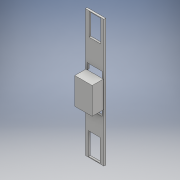
# Autodesk Inventor part: Base_trem
Saved by Autodesk Inventor 2018 (Build 220112000, 112)
## iProperties
Created: 2018-02-24
Part Number: Base_trem
Material: Generic
Document SubType Name: Modeling
Designer: matheus
Density: 1 g/cm^3
Appearance: Default
Author: matheus
Autodesk Inventor part; units mm, degrees
ref_plane "YZ Plane" through (0, 0, 0) normal (1, 0, 0) x (0, 1, 0)
ref_plane "XZ Plane" through (0, 0, 0) normal (0, 1, 0) x (-1, 0, 0)
ref_plane "XY Plane" through (0, 0, 0) normal (0, 0, 1) x (1, 0, 0)
sketch "Sketch1" plane through (0, 0, 0) normal (0, 1, 0) x (-1, 0, 0)
  line L0 (-15, 102.5) -> (15, 102.5)
  line L1 (15, 102.5) -> (15, -102.5)
  line L2 (15, -102.5) -> (-15, -102.5)
  line L3 (-15, -102.5) -> (-15, 102.5)
  point P0 (0, 0)
  constraints: 8 end point, 2 parallel, 1 horizontal, 1 perpendicular
extrude "Extrusion1" add sketch "Sketch1" along normal blind 3
sketch "Sketch2" plane through (0, 0, 0) normal (0, -1, 0) x (1, 0, 0)
  line L0 (-15, -102.5) -> (-15, 102.5) projected
  line L1 (-15, -102.5) -> (-15, -101.5)
  line L2 (-10, -101.5) -> (9, -101.5)
  line L3 (9, -101.5) -> (9, -65.5)
  line L4 (9, -65.5) -> (-10, -65.5)
  line L5 (-10, -65.5) -> (-10, -101.5)
  point P0 (0, 0)
  dimension "d7" = 5
  dimension "d8" = 19
  dimension "d9" = 36
  constraints: 10 end point, 2 parallel, 1 horizontal, 1 perpendicular, 1 point on line
  measures "d7" distance of L1.end L2.start
  measures "d8" distance of L4.end L3.end
  measures "d9" distance of L3.end L2.end
extrude "Extrusion2" cut sketch "Sketch2" against normal through all
sketch "Sketch3" plane through (0, 3, 0) normal (0, 1, 0) x (1, 0, 0)
  line L0 (15, 102.5) -> (-15, 102.5) projected
  line L1 (15, -102.5) -> (15, 102.5) projected
  line L2 (7, 47.5) -> (-8, 47.5)
  line L3 (-8, 47.5) -> (-8, -52.5)
  line L4 (-8, -52.5) -> (7, -52.5)
  line L5 (7, -52.5) -> (7, 47.5)
  point P0 (0, 0)
  dimension "d14" = 15
  dimension "d15" = 100
  constraints: 8 end point, 2 parallel, 1 horizontal, 1 perpendicular
  measures "d14" distance of L4.end L3.end
  measures "d15" distance of L2.end L3.end
extrude "Extrusion3" cut sketch "Sketch3" against normal through all
sketch "Sketch4" plane through (0, 3, 0) normal (0, 1, 0) x (1, 0, 0)
  line L0 (-15, -102.5) -> (15, -102.5) projected
  line L1 (10, -101.5) -> (-9, -101.5)
  line L2 (-9, -101.5) -> (-9, -65.5)
  line L3 (-9, -65.5) -> (10, -65.5)
  line L4 (10, -65.5) -> (10, -101.5)
  point P0 (0, 0)
  dimension "d20" = 19
  dimension "d21" = 36
  constraints: 8 end point, 2 parallel, 1 horizontal, 1 perpendicular
  measures "d20" distance of L2.end L3.end
  measures "d21" distance of L1.end L2.end
extrude "Extrusion4" cut sketch "Sketch4" against normal through all
sketch "Sketch5" plane through (0, 0, 0) normal (0, -1, 0) x (1, 0, 0)
  line L0 (7, 52.5) -> (7, -47.5) projected
  line L1 (-8, -47.5) -> (-8, 52.5) projected
  line L2 (7, 52.5) -> (-8, 52.5)
  line L3 (-8, 52.5) -> (-8, -47.5)
  line L4 (-8, -47.5) -> (7, -47.5)
  line L5 (7, -47.5) -> (7, 52.5)
  point P0 (0, 0)
  constraints: 8 end point, 2 parallel, 1 horizontal, 1 perpendicular
extrude "Extrusion5" add sketch "Sketch5" against normal blind 3
sketch "Sketch6" plane through (0, 0, 0) normal (0, -1, 0) x (1, 0, 0)
  line L0 (15, -102.5) -> (-15, -102.5) projected
  line L1 (12, -34.5) -> (12, -24.5)
  line L2 (15, 102.5) -> (15, -102.5) projected
  line L3 (12, 18.5) -> (12, 28.5)
  line L4 (-15, -102.5) -> (-15, 102.5) projected
  line L5 (12, -24.5) -> (14, -24.5)
  line L6 (14, -24.5) -> (14, 18.5)
  line L7 (14, 18.5) -> (12, 18.5)
  line L8 (12, 28.5) -> (-12, 28.5)
  line L9 (-12, 28.5) -> (-12, 18.5)
  line L10 (-12, 18.5) -> (-14, 18.5)
  line L11 (-14, 18.5) -> (-14, -24.5)
  line L12 (-14, -24.5) -> (-12, -24.5)
  line L13 (-12, -24.5) -> (-12, -34.5)
  line L14 (-12, -34.5) -> (12, -34.5)
  point P0 (0, 0)
  dimension "d32" = 10
  dimension "d36" = 2
  dimension "d39" = 24
  dimension "d40" = 10
  dimension "d41" = 2
  dimension "d42" = 43
  dimension "d43" = 2
  constraints: 24 end point, 5 perpendicular, 4 point on line, 2 horizontal, 1 parallel
  measures "d32" distance of L3.start L3.end
  measures "d36" distance of L1.end L5.end
  measures "d39" distance of L3.end L8.end
  measures "d40" distance of L8.end L9.end
  measures "d41" distance of L9.end L10.end
  measures "d42" distance of L10.end L11.end
  measures "d43" distance of L11.end L12.end
extrude "Extrusion6" cut sketch "Sketch6" against normal through all
sketch "Sketch7" plane through (0, 0, 0) normal (0, -1, 0) x (1, 0, 0)
  line L0 (-14, 18.5) -> (-14, -24.5) projected
  line L1 (14, -24.5) -> (14, 18.5) projected
  line L2 (-14, 18.5) -> (14, 18.5)
  line L3 (14, 18.5) -> (14, -24.5)
  line L4 (14, -24.5) -> (-14, -24.5)
  line L5 (-14, -24.5) -> (-14, 18.5)
  point P0 (0, 0)
  constraints: 8 end point, 2 parallel, 1 horizontal, 1 perpendicular
extrude "Extrusion7" add sketch "Sketch7" along normal blind 18
shell "Shell1" thickness 1 removed faces 1 at (-4, 0, -10.1667)
body "Solid1"
